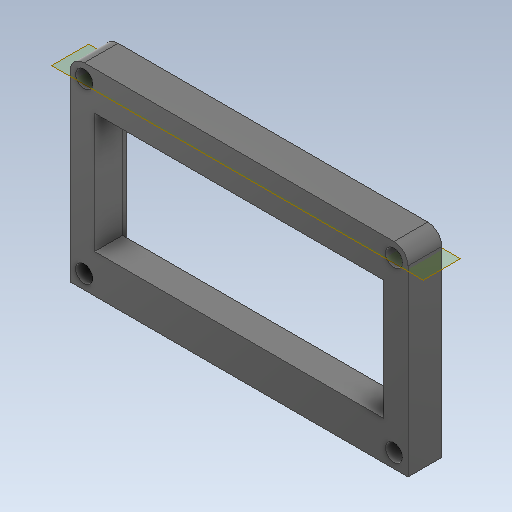
# Autodesk Inventor part: Faceplate
Saved by Autodesk Inventor 2020 (Build 240168000, 168)
## iProperties
Created: 2020-04-16
Part Number: Faceplate
Material: Generic
Document SubType Name: Modeling
Designer: amsmi
Density: 1 g/cm^3
Appearance: Default
Author: amsmi
Autodesk Inventor part; units mm, degrees
ref_plane "YZ Plane" through (0, 0, 0) normal (1, 0, 0) x (0, 1, 0)
ref_plane "XZ Plane" through (0, 0, 0) normal (0, 1, 0) x (-1, 0, 0)
sketch "Sketch1" plane through (0, 0, 0) normal (0, 0, 1) x (1, 0, 0)
  line L0 (57.15, -33.2867) -> (-57.15, -33.2867)
  line L1 (-57.15, -33.2867) -> (-57.15, 33.2867)
  line L2 (-57.15, 33.2867) -> (57.15, 33.2867)
  line L3 (57.15, 33.2867) -> (57.15, -33.2867)
  line L4 (57.15, -33.2867) -> (-57.15, 33.2867) construction
  line L5 (-57.15, -33.2867) -> (57.15, 33.2867) construction
  point P0 (0, 0)
  dimension "d2" = 114.3
  dimension "d3" = 66.5734
  constraints: 12 end point, 2 midpoint, 2 parallel, 1 horizontal, 1 perpendicular
  measures "d2" distance of L1.end L2.end
  measures "d3" distance of L0.end L1.end
extrude "Extrusion1" add sketch "Sketch1" along normal blind 11.43
sketch "Sketch5" plane through (0, 0, 11.43) normal (0, 0, 1) x (1, 0, 0)
  circle A0 centre (-52.3875, 28.5242) radius 1.4478 projected
  circle A1 centre (52.3875, 28.5242) radius 1.4478 projected
  circle A2 centre (52.3875, -28.5242) radius 1.4478 projected
  circle A3 centre (-52.3875, -28.5242) radius 1.4478 projected
  point P0 (0, 0)
  constraints: 4 coincident
hole "Hole2" at (-52.3875, -28.5242, 11.43) at (-52.3875, 28.5242, 11.43) at (52.3875, 28.5242, 11.43) at (52.3875, -28.5242, 11.43) direction (0, 0, -1) diameter 3.2766 end through all counterbore diameter 5.842 counterbore depth 9.525 clearance for "Socket Head Cap Screw" size "#4" standard "Ansi Unified Screw Threads"
fillet "Fillet1" radius 4.7625 2 edges at (-57.15, 33.2867, 5.715) (57.15, 33.2867, 5.715)
sketch "Sketch3" plane through (0, 0, 0) normal (0, 0, -1) x (-1, 0, 0)
  line L0 (49.0474, 30.1117) -> (-49.0474, 30.1117) projected
  line L1 (-49.0474, 30.1117) -> (-49.0474, -30.1117) projected
  line L2 (49.0474, -30.1117) -> (49.0474, 30.1117) projected
  line L3 (-49.0474, -30.1117) -> (49.0474, -30.1117) projected
  line L4 (-49.5554, 30.6197) -> (49.5554, 30.6197)
  line L5 (49.5554, 30.6197) -> (49.5554, -30.6197)
  line L6 (49.5554, -30.6197) -> (-49.5554, -30.6197)
  line L7 (-49.5554, -30.6197) -> (-49.5554, 30.6197)
  point P0 (0, 0)
  dimension "d23" = 0.508
  constraints: 8 end point, 3 other
  measures "d23" distance between parallel lines of L0 L4
ref_plane "Work Plane1" through (-49.0474, -30.1117, 1.9812) normal (0, 0, 1) x (1, 0, 0)
extrude "Extrusion4" cut sketch "Sketch3" against normal up to surface (1.9812 mm away) contours L2 L3 L1 L0 | L4 L5 L6 L7
sketch "Sketch6" plane through (49.5554, 30.6197, 1.9812) normal (0, 0, -1) x (-1, 0, 0)
  line L0 (1.016, -10.7188) -> (98.0948, -10.7188) projected
  line L1 (98.0948, -50.5206) -> (1.016, -50.5206) projected
  line L2 (98.0948, -10.7188) -> (1.016, -10.7188)
  line L3 (1.016, -10.7188) -> (1.016, -50.5206)
  line L4 (1.016, -50.5206) -> (98.0948, -50.5206)
  line L5 (98.0948, -50.5206) -> (98.0948, -10.7188)
  line L6 (0.635, -50.9016) -> (0.635, -10.3378)
  line L7 (0.635, -10.3378) -> (98.4758, -10.3378)
  line L8 (98.4758, -10.3378) -> (98.4758, -50.9016)
  line L9 (98.4758, -50.9016) -> (0.635, -50.9016)
  point P0 (49.5554, -30.6197)
  dimension "d26" = 0.381
  constraints: 16 end point, 4 parallel, 2 perpendicular, 1 horizontal, 3 other
  measures "d26" distance between parallel lines of L3 L6
extrude "Extrusion5" cut sketch "Sketch6" against normal through all contours L0 L5 L1 L3 | L6 L7 L8 L9
sketch "Sketch7" plane through (49.5554, 30.6197, 1.9812) normal (0, 0, -1) x (-1, 0, 0)
  line L0 (47.898, 0) -> (90.57, 0)
  line L1 (90.57, 0) -> (90.57, -10.3378)
  line L2 (90.57, -10.3378) -> (47.898, -10.3378)
  line L3 (47.898, -10.3378) -> (47.898, 0)
  line L4 (48.914, -2.2542) -> (48.914, -3.7782) projected
  line L5 (89.554, -3.7782) -> (89.554, -2.2542) projected
  line L6 (87.522, -4.2862) -> (89.046, -4.2862) projected
  line L7 (0, 0) -> (99.1108, 0) projected
  line L8 (0.635, -10.3378) -> (98.4758, -10.3378) projected
  point P0 (49.5554, -30.6197)
  dimension "d29" = 1.016
  dimension "d30" = 1.016
  constraints: 8 end point, 2 parallel, 2 point on line, 1 horizontal, 1 perpendicular
  measures "d29" distance between parallel lines of L1 L5
  measures "d30" distance between parallel lines of L3 L4
extrude "Extrusion6" cut sketch "Sketch7" against normal blind 5.08
sketch "Sketch8" plane through (49.5554, -30.6197, 1.9812) normal (0, 0, -1) x (-1, 0, 0)
  circle A0 centre (73.7616, 21.2344) radius 5.0165 construction
  circle A1 centre (36.83, 38.2524) radius 5.0165 construction
  circle A2 centre (22.4028, 29.7434) radius 5.0165 construction
  circle A3 centre (44.958, 21.6408) radius 5.0165 construction
  circle A4 centre (66.4464, 37.5158) radius 5.0165 construction
  line L0 (63.7286, 13.634) -> (64.3364, 14.2474) construction
  line L1 (64.3364, 14.2474) -> (67.945, 10.6719) construction
  line L2 (67.945, 10.6719) -> (67.3372, 10.0584) construction
  line L3 (67.3372, 10.0584) -> (63.7286, 13.634) construction
  line L4 (95.8995, 51.3588) -> (96.5073, 50.7453) construction
  line L5 (96.5073, 50.7453) -> (92.8987, 47.1698) construction
  line L6 (92.8987, 47.1698) -> (92.2909, 47.7832) construction
  line L7 (92.2909, 47.7832) -> (95.8995, 51.3588) construction
  line L8 (35.2425, 47.7832) -> (34.6347, 47.1698) construction
  line L9 (34.6347, 47.1698) -> (31.0261, 50.7453) construction
  line L10 (31.0261, 50.7453) -> (31.6339, 51.3588) construction
  line L11 (31.6339, 51.3588) -> (35.2425, 47.7832) construction
  line L12 (6.8199, 47.7832) -> (6.2121, 47.1698) construction
  line L13 (6.2121, 47.1698) -> (2.6035, 50.7453) construction
  line L14 (2.6035, 50.7453) -> (3.2113, 51.3588) construction
  line L15 (3.2113, 51.3588) -> (6.8199, 47.7832) construction
  line L16 (6.3518, 14.2474) -> (6.9596, 13.634) construction
  line L17 (6.9596, 13.634) -> (3.351, 10.0584) construction
  line L18 (3.351, 10.0584) -> (2.7432, 10.6719) construction
  line L19 (2.7432, 10.6719) -> (6.3518, 14.2474) construction
  line L20 (35.3822, 13.634) -> (31.7736, 10.0584) construction
  line L21 (31.7736, 10.0584) -> (31.1658, 10.6719) construction
  line L22 (31.1658, 10.6719) -> (34.7744, 14.2474) construction
  line L23 (34.7744, 14.2474) -> (35.3822, 13.634) construction
  line L24 (92.759, 14.2474) -> (96.3676, 10.6719) construction
  line L25 (96.3676, 10.6719) -> (95.7598, 10.0584) construction
  line L26 (95.7598, 10.0584) -> (92.1512, 13.634) construction
  line L27 (92.1512, 13.634) -> (92.759, 14.2474) construction
  line L28 (67.4769, 51.3588) -> (68.0847, 50.7453) construction
  line L29 (68.0847, 50.7453) -> (64.4761, 47.1698) construction
  line L30 (64.4761, 47.1698) -> (63.8683, 47.7832) construction
  line L31 (63.8683, 47.7832) -> (67.4769, 51.3588) construction
  line L32 (51.689, 60.4774) -> (53.7718, 60.4774) construction
  line L33 (53.7718, 60.4774) -> (53.7718, 58.2168) construction
  arc A5 (51.689, 58.2168) -> (53.7718, 58.2168) centre (52.7304, 58.2168) ccw construction
  line L34 (51.689, 58.2168) -> (51.689, 60.4774) construction
  line L35 (56.769, 60.4774) -> (58.8518, 60.4774) construction
  line L36 (58.8518, 60.4774) -> (58.8518, 58.2168) construction
  arc A6 (56.769, 58.2168) -> (58.8518, 58.2168) centre (57.8104, 58.2168) ccw construction
  line L37 (56.769, 58.2168) -> (56.769, 60.4774) construction
  line L38 (61.849, 60.4774) -> (63.9318, 60.4774) construction
  line L39 (63.9318, 60.4774) -> (63.9318, 58.2168) construction
  arc A7 (61.849, 58.2168) -> (63.9318, 58.2168) centre (62.8904, 58.2168) ccw construction
  line L40 (61.849, 58.2168) -> (61.849, 60.4774) construction
  line L41 (66.929, 60.4774) -> (69.0118, 60.4774) construction
  line L42 (69.0118, 60.4774) -> (69.0118, 58.2168) construction
  arc A8 (66.929, 58.2168) -> (69.0118, 58.2168) centre (67.9704, 58.2168) ccw construction
  line L43 (66.929, 58.2168) -> (66.929, 60.4774) construction
  line L44 (72.009, 60.4774) -> (74.0918, 60.4774) construction
  line L45 (74.0918, 60.4774) -> (74.0918, 58.2168) construction
  arc A9 (72.009, 58.2168) -> (74.0918, 58.2168) centre (73.0504, 58.2168) ccw construction
  line L46 (72.009, 58.2168) -> (72.009, 60.4774) construction
  line L47 (77.089, 60.4774) -> (79.1718, 60.4774) construction
  line L48 (79.1718, 60.4774) -> (79.1718, 58.2168) construction
  arc A10 (77.089, 58.2168) -> (79.1718, 58.2168) centre (78.1304, 58.2168) ccw construction
  line L49 (77.089, 58.2168) -> (77.089, 60.4774) construction
  line L50 (82.169, 60.4774) -> (84.2518, 60.4774) construction
  line L51 (84.2518, 60.4774) -> (84.2518, 58.2168) construction
  arc A11 (82.169, 58.2168) -> (84.2518, 58.2168) centre (83.2104, 58.2168) ccw construction
  line L52 (82.169, 58.2168) -> (82.169, 60.4774) construction
  line L53 (87.249, 60.4774) -> (89.3318, 60.4774) construction
  line L54 (89.3318, 60.4774) -> (89.3318, 58.2168) construction
  arc A12 (87.249, 58.2168) -> (89.3318, 58.2168) centre (88.2904, 58.2168) ccw construction
  line L55 (87.249, 58.2168) -> (87.249, 60.4774) construction
  line L56 (84.709, 60.4774) -> (86.7918, 60.4774) construction
  line L57 (86.7918, 60.4774) -> (86.7918, 58.2168) construction
  arc A13 (84.709, 58.2168) -> (86.7918, 58.2168) centre (85.7504, 58.2168) ccw construction
  line L58 (84.709, 58.2168) -> (84.709, 60.4774) construction
  line L59 (79.629, 60.4774) -> (81.7118, 60.4774) construction
  line L60 (81.7118, 60.4774) -> (81.7118, 58.2168) construction
  arc A14 (79.629, 58.2168) -> (81.7118, 58.2168) centre (80.6704, 58.2168) ccw construction
  line L61 (79.629, 58.2168) -> (79.629, 60.4774) construction
  line L62 (74.549, 60.4774) -> (76.6318, 60.4774) construction
  line L63 (76.6318, 60.4774) -> (76.6318, 58.2168) construction
  arc A15 (74.549, 58.2168) -> (76.6318, 58.2168) centre (75.5904, 58.2168) ccw construction
  line L64 (74.549, 58.2168) -> (74.549, 60.4774) construction
  line L65 (69.469, 60.4774) -> (71.5518, 60.4774) construction
  line L66 (71.5518, 60.4774) -> (71.5518, 58.2168) construction
  arc A16 (69.469, 58.2168) -> (71.5518, 58.2168) centre (70.5104, 58.2168) ccw construction
  line L67 (69.469, 58.2168) -> (69.469, 60.4774) construction
  line L68 (64.389, 60.4774) -> (66.4718, 60.4774) construction
  line L69 (66.4718, 60.4774) -> (66.4718, 58.2168) construction
  arc A17 (64.389, 58.2168) -> (66.4718, 58.2168) centre (65.4304, 58.2168) ccw construction
  line L70 (64.389, 58.2168) -> (64.389, 60.4774) construction
  line L71 (59.309, 60.4774) -> (61.3918, 60.4774) construction
  line L72 (61.3918, 60.4774) -> (61.3918, 58.2168) construction
  arc A18 (59.309, 58.2168) -> (61.3918, 58.2168) centre (60.3504, 58.2168) ccw construction
  line L73 (59.309, 58.2168) -> (59.309, 60.4774) construction
  line L74 (54.229, 60.4774) -> (56.3118, 60.4774) construction
  line L75 (56.3118, 60.4774) -> (56.3118, 58.2168) construction
  arc A19 (54.229, 58.2168) -> (56.3118, 58.2168) centre (55.2704, 58.2168) ccw construction
  line L76 (54.229, 58.2168) -> (54.229, 60.4774) construction
  line L77 (49.149, 60.4774) -> (51.2318, 60.4774) construction
  line L78 (51.2318, 60.4774) -> (51.2318, 58.2168) construction
  arc A20 (49.149, 58.2168) -> (51.2318, 58.2168) centre (50.1904, 58.2168) ccw construction
  line L79 (49.149, 58.2168) -> (49.149, 60.4774) construction
  circle A21 centre (3.0734, 58.1152) radius 2.4892 construction
  circle A22 centre (96.0374, 58.1152) radius 2.4892 construction
  circle A23 centre (96.0374, 3.1242) radius 2.4892 construction
  circle A24 centre (3.0734, 3.1242) radius 2.4892 construction
  line L80 (0.508, 0.508) -> (98.6028, 0.508) construction
  line L81 (98.6028, 0.508) -> (98.6028, 60.7314) construction
  line L82 (98.6028, 60.7314) -> (0.508, 60.7314) construction
  line L83 (0.508, 60.7314) -> (0.508, 0.508) construction
  point P0 (49.5554, 30.6197)
  constraints: 4 coincident
hole "Hole3" at (46.482, 27.4955, 1.9812) at (-46.482, 27.4955, 1.9812) at (-46.482, -27.4955, 1.9812) at (46.482, -27.4955, 1.9812) direction (0, 0, 1) diameter 2.2606 depth 6.35
chamfer "Chamfer1" distance 0.3175 angle 45 4 edges at (46.482, 26.3652, 1.9812) (46.482, -28.6258, 1.9812) (-46.482, -28.6258, 1.9812) (-46.482, 26.3652, 1.9812)
ref_plane "Work Plane2" through (46.482, 27.4955, 1.9812) normal (0, -1, 0) x (1, 0, 0)
sketch "Sketch9" plane through (46.482, 27.4955, 1.9812) normal (0, -1, 0) x (1, 0, 0)
  line L0 (-1.1303, 6.35) -> (-1.1303, 6.8263)
  line L1 (-1.1303, 6.8263) -> (-1.4053, 6.6675)
  line L2 (-1.4053, 6.6675) -> (-1.4053, 6.5088)
  line L3 (-1.4053, 6.5088) -> (-1.1303, 6.35)
  line L4 (-1.1303, 6.35) -> (1.1303, 6.35) projected
  line L5 (1.4478, 0) -> (1.1303, 0.3175) projected
  line L6 (0, 6.35) -> (0, 0)
  point P0 (-46.482, -1.9812)
  dimension "d43" = 60
  dimension "d44" = 0.4763
  dimension "d45" = 0.1588
  dimension "d46" = 6.8262
  constraints: 10 end point, 2 vertical, 1 equal length, 1 midpoint, 1 parallel
  measures "d43" angle of L1 L3
  measures "d44" distance of L0.start L0.end
  measures "d45" distance of L1.end L2.end
  measures "d46" vertical distance of L0.end L5.start
coil "Coil1" sketch "Sketch9" operation cut axis through (46.482, 27.4955, 8.3312) along (0, 0, -1) pitch 0.635 turns 10.75 hand right
pattern_sketch "Sketch Driven Pattern1" of "Coil1" from (46.482, 27.4955, 1.9812) copies at (-46.482, 27.4955, 1.9812) at (-46.482, -27.4955, 1.9812) at (46.482, -27.4955, 1.9812)
equation "\"d45\" = 0.333333 * d44"
equation "\"d48\" = d46"
body "Solid1"
